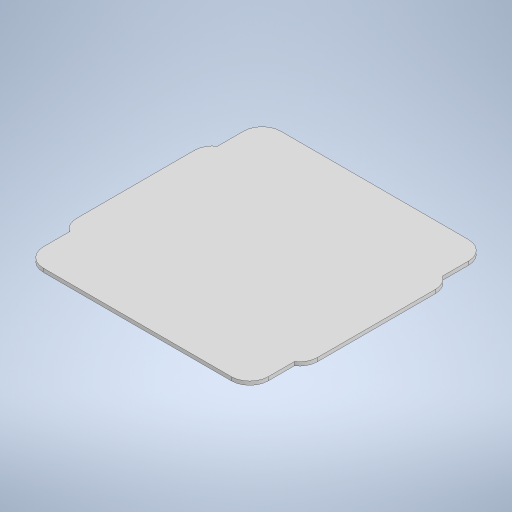
# Autodesk Inventor part: Part2
Saved by Autodesk Inventor 2024.2 (Build 282272000, 272)
## iProperties
Created: 2024-01-05
Part Number: Part2
Material: Generic
Document SubType Name: Modeling
Designer: rohan
Density: 1 g/cm^3
Appearance: Default
Author: rohan
Autodesk Inventor part; units mm, degrees
ref_plane "YZ Plane" through (0, 0, 0) normal (1, 0, 0) x (0, 1, 0)
ref_plane "XZ Plane" through (0, 0, 0) normal (0, 1, 0) x (-1, 0, 0)
ref_plane "XY Plane" through (0, 0, 0) normal (0, 0, 1) x (1, 0, 0)
sketch "Sketch1" plane through (0, 0, 0) normal (0, 1, 0) x (-1, 0, 0)
  line L0 (-81.1911, 89.7001) -> (81.1911, 89.7001)
  line L1 (84.3661, 86.5251) -> (84.3661, 57.1881)
  line L2 (81.1911, -89.7001) -> (-81.1911, -89.7001)
  line L3 (-84.3661, 89.7001) -> (84.3661, -89.7001) construction
  line L4 (84.3661, 89.7001) -> (-84.3661, -89.7001) construction
  line L5 (88.0999, 54.0131) -> (87.5411, 54.0131)
  line L6 (87.5411, -54.0131) -> (88.0999, -54.0131)
  line L7 (91.2749, -50.8381) -> (91.2749, 50.8381)
  arc A0 (84.3661, 57.1881) -> (87.5411, 54.0131) centre (87.5411, 57.1881) ccw
  arc A1 (91.2749, 50.8381) -> (88.0999, 54.0131) centre (88.0999, 50.8381) ccw
  arc A2 (88.0999, -54.0131) -> (91.2749, -50.8381) centre (88.0999, -50.8381) ccw
  line L8 (84.3661, -57.1881) -> (84.3661, -86.5251)
  arc A3 (87.5411, -54.0131) -> (84.3661, -57.1881) centre (87.5411, -57.1881) ccw
  arc A4 (84.3661, 86.5251) -> (81.1911, 89.7001) centre (81.1911, 86.5251) ccw
  arc A5 (-81.1911, 89.7001) -> (-84.3661, 86.5251) centre (-81.1911, 86.5251) ccw
  arc A6 (-84.3661, -86.5251) -> (-81.1911, -89.7001) centre (-81.1911, -86.5251) ccw
  arc A7 (81.1911, -89.7001) -> (84.3661, -86.5251) centre (81.1911, -86.5251) ccw
  line L9 (0, 113.6311) -> (0, -138.756)
  line L10 (-91.2749, -50.8381) -> (-91.2749, 50.8381)
  arc A8 (-87.5411, 54.0131) -> (-84.3661, 57.1881) centre (-87.5411, 57.1881) ccw
  arc A9 (-91.2749, -50.8381) -> (-88.0999, -54.0131) centre (-88.0999, -50.8381) ccw
  arc A10 (-84.3661, -57.1881) -> (-87.5411, -54.0131) centre (-87.5411, -57.1881) ccw
  line L11 (-84.3661, -86.5251) -> (-84.3661, -57.1881)
  line L12 (-84.3661, 57.1881) -> (-84.3661, 86.5251)
  arc A11 (-88.0999, 54.0131) -> (-91.2749, 50.8381) centre (-88.0999, 50.8381) ccw
  line L13 (-88.0999, 54.0131) -> (-87.5411, 54.0131)
  line L14 (-88.0999, -54.0131) -> (-87.5411, -54.0131)
  point P0 (0, 0)
  point P1 (84.3661, -54.0131)
  point P2 (91.2749, -54.0131)
  point P3 (84.3661, 71.8566)
  dimension "d0" = 168.7322
  dimension "d1" = 179.4002
  dimension "d2" = 6.9088
  dimension "d4" = 3.175
  dimension "d5" = 3.175
  dimension "d6" = 3.175
  constraints: 30 end point, 24 point on circle, 18 tangent, 12 centre point, 12 point on line, 12 symmetric about line, 5 equal radius, 4 horizontal, 4 parallel, 3 midpoint, 2 perpendicular, 1 vertical, 4 other
  measures "d0" distance of L3.end L4.end
  measures "d1" distance of L4.start L3.end
  measures "d2" distance of point (91.275, -54.013) point (84.366, -54.013)
  measures "d4" radius of A0
  measures "d5" radius of A3
  measures "d6" radius of A4
extrude "Extrusion1" add sketch "Sketch1" along normal blind 3.175
sketch "Sketch2" plane through (0, 3.175, 0) normal (0, 1, 0) x (1, 0, 0)
  line L0 (-81.1911, -89.7001) -> (81.1911, -89.7001) projected
  arc A0 (81.1911, -89.7001) -> (84.3661, -86.5251) centre (81.1911, -86.5251) ccw projected
  line L1 (84.3661, -86.5251) -> (84.3661, -57.1881) projected
  arc A1 (87.5411, -54.0131) -> (84.3661, -57.1881) centre (87.5411, -57.1881) ccw projected
  line L2 (87.5411, -54.0131) -> (88.0999, -54.0131) projected
  arc A2 (88.0999, -54.0131) -> (91.2749, -50.8381) centre (88.0999, -50.8381) ccw projected
  line L3 (91.2749, -50.8381) -> (91.2749, 50.8381) projected
  arc A3 (91.2749, 50.8381) -> (88.0999, 54.0131) centre (88.0999, 50.8381) ccw projected
  line L4 (88.0999, 54.0131) -> (87.5411, 54.0131) projected
  arc A4 (84.3661, 57.1881) -> (87.5411, 54.0131) centre (87.5411, 57.1881) ccw projected
  line L5 (84.3661, 57.1881) -> (84.3661, 86.5251) projected
  arc A5 (84.3661, 86.5251) -> (81.1911, 89.7001) centre (81.1911, 86.5251) ccw projected
  line L6 (81.1911, 89.7001) -> (-81.1911, 89.7001) projected
  arc A6 (-81.1911, 89.7001) -> (-84.3661, 86.5251) centre (-81.1911, 86.5251) ccw projected
  line L7 (-84.3661, 86.5251) -> (-84.3661, 57.1881) projected
  arc A7 (-87.5411, 54.0131) -> (-84.3661, 57.1881) centre (-87.5411, 57.1881) ccw projected
  line L8 (-87.5411, 54.0131) -> (-88.0999, 54.0131) projected
  arc A8 (-88.0999, 54.0131) -> (-91.2749, 50.8381) centre (-88.0999, 50.8381) ccw projected
  line L9 (-91.2749, 50.8381) -> (-91.2749, -50.8381) projected
  arc A9 (-91.2749, -50.8381) -> (-88.0999, -54.0131) centre (-88.0999, -50.8381) ccw projected
  line L10 (-88.0999, -54.0131) -> (-87.5411, -54.0131) projected
  arc A10 (-84.3661, -57.1881) -> (-87.5411, -54.0131) centre (-87.5411, -57.1881) ccw projected
  line L11 (-84.3661, -57.1881) -> (-84.3661, -86.5251) projected
  arc A11 (-84.3661, -86.5251) -> (-81.1911, -89.7001) centre (-81.1911, -86.5251) ccw projected
  line L12 (-81.1911, -102.4001) -> (81.1911, -102.4001)
  line L13 (-103.9749, -50.8381) -> (-103.9749, 50.8381)
  line L14 (-97.0661, 63.9386) -> (-97.0661, 86.5251)
  line L15 (-81.1911, 102.4001) -> (81.1911, 102.4001)
  line L16 (97.0661, -86.5304) -> (97.0661, -63.9386)
  line L17 (103.9749, -50.8381) -> (103.9749, 50.8381)
  line L18 (97.0661, 63.9386) -> (97.0661, 86.5251)
  line L19 (-97.0661, -86.5251) -> (-97.0661, -63.9386)
  arc A12 (81.1911, -102.4001) -> (97.0661, -86.5251) centre (81.1911, -86.5251) ccw
  arc A13 (97.0661, -63.9386) -> (103.9749, -50.8381) centre (88.0999, -50.8381) ccw
  arc A14 (103.9749, 50.8381) -> (97.0661, 63.9386) centre (88.0999, 50.8381) ccw
  arc A15 (97.0661, 86.5251) -> (81.1911, 102.4001) centre (81.1911, 86.5251) ccw
  arc A16 (-81.1911, 102.4001) -> (-97.0661, 86.5251) centre (-81.1911, 86.5251) ccw
  arc A17 (-97.0661, 63.9386) -> (-103.9749, 50.8381) centre (-88.0999, 50.8381) ccw
  arc A18 (-103.9749, -50.8381) -> (-97.0661, -63.9386) centre (-88.0999, -50.8381) ccw
  arc A19 (-97.0661, -86.5251) -> (-81.1911, -102.4001) centre (-81.1911, -86.5251) ccw
  point P0 (0, 0)
  point P1 (84.3661, -71.8566)
  dimension "d9" = 12.7
  dimension "d10" = 12.7
  dimension "d11" = 12.7
  dimension "d12" = 12.7
  dimension "d13" = 12.7
  dimension "d14" = 12.7
  dimension "d15" = 12.7
  dimension "d16" = 12.7
  constraints: 17 point on circle, 16 end point, 8 centre point, 8 coincident, 6 vertical, 2 horizontal, 2 point on line, 1 midpoint, 1 tangent
  measures "d9" distance between parallel lines of L12 L0
  measures "d10" distance between parallel lines of L11 L19
  measures "d11" distance between parallel lines of L13 L9
  measures "d12" distance between parallel lines of L14 L7
  measures "d13" distance between parallel lines of L15 L6
  measures "d14" distance between parallel lines of L5 L18
  measures "d15" distance between parallel lines of L3 L17
  measures "d16" distance from line of point (84.366, -71.857) L16
extrude "Extrusion2" add sketch "Sketch2" against normal up to surface (3.175 mm away)
body "Solid1"
